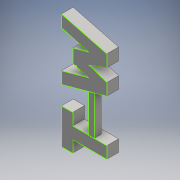
# Autodesk Inventor part: hw1-initials
Saved by Autodesk Inventor 2016 SP1 (Build 200210100, 210)
## iProperties
Created: 2016-01-28
Part Number: hw1-initials
Material: Generic
Document SubType Name: Modeling
Designer: Wes
Density: 1 g/cm^3
Appearance: Default
Author: Wes
Autodesk Inventor part; units mm, degrees
ref_plane "YZ Plane" through (0, 0, 0) normal (1, 0, 0) x (0, 1, 0)
ref_plane "XZ Plane" through (0, 0, 0) normal (0, 1, 0) x (-1, 0, 0)
ref_plane "XY Plane" through (0, 0, 0) normal (0, 0, 1) x (1, 0, 0)
sketch "Sketch1" plane through (0, 0, 0) normal (0, 1, 0) x (-1, 0, 0)
  line L0 (6.2763, 15.9249) -> (6.2763, 10.9249)
  line L1 (6.2763, 10.9249) -> (-5.2771, 7.6502)
  line L2 (-5.2771, 7.6502) -> (1.4843, 5.8136)
  line L3 (1.4843, 5.8136) -> (1.4843, 0.1561)
  line L4 (1.4843, 0.1561) -> (-5.2771, -1.7603)
  line L5 (-5.2771, -1.7603) -> (6.2763, -4.934)
  line L6 (6.2763, -4.934) -> (6.2763, -9.934)
  line L7 (6.2763, -9.934) -> (-13.0093, -4.6363)
  line L8 (-13.0093, -4.6363) -> (-13.0093, 0.3637)
  line L9 (-13.0093, 0.3637) -> (-5.2771, 2.9849)
  line L10 (-5.2771, 2.9849) -> (-13.0093, 5.8136)
  line L11 (-13.0093, 5.8136) -> (-13.0093, 10.9249)
  line L12 (-13.0093, 10.9249) -> (6.2763, 15.9249)
  line L13 (6.2763, -17.865) -> (6.2763, -32.865)
  line L14 (6.2763, -32.865) -> (1.4843, -32.865)
  line L15 (1.4843, -32.865) -> (1.4843, -27.865)
  line L16 (1.4843, -27.865) -> (-13.0093, -27.865)
  line L17 (-13.0093, -27.865) -> (-13.0093, -22.865)
  line L18 (-13.0093, -22.865) -> (1.4843, -22.865)
  line L19 (1.4843, -22.865) -> (1.4843, -17.865)
  line L20 (1.4843, -17.865) -> (6.2763, -17.865)
  line L21 (-5.2771, -6.7603) -> (-5.2771, -22.865)
  line L22 (-7.6463, -22.865) -> (-7.6463, -6.1095)
  point P0 (0, 0)
  constraints: 46 end point, 9 point on line, 7 perpendicular, 5 parallel, 3 vertical
extrude "Extrusion1" add sketch "Sketch1" along normal blind 5 contours L0 L1 L2 L3 L4 L5 L6 L7 L8 L9 L10 L11 L12 | L18 L19 L20 L13 L14 L15 L16 L17
extrude "Extrusion2" add sketch "Sketch1" along normal blind 3 contours L7 L21 L18 L22
body "Solid1"
